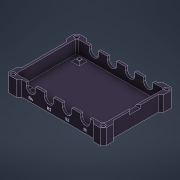
# Autodesk Inventor part: Case
Saved by Autodesk Inventor 2021.4 (Build 254397000, 397)
## iProperties
Created: 2022-02-15
Part Number: Case
Material: Generic
Document SubType Name: Modeling
Designer: Alex
Density: 1 g/cm^3
Appearance: Default
Author: Alex
Autodesk Inventor part; units mm, degrees
note: some values were not read from the file. Chosen so that the rebuilt part matches the saved one: direction of "Emboss1"; direction of "Emboss2".
ref_plane "YZ Plane" through (0, 0, 0) normal (1, 0, 0) x (0, 1, 0)
ref_plane "XZ Plane" through (0, 0, 0) normal (0, 1, 0) x (-1, 0, 0)
ref_plane "XY Plane" through (0, 0, 0) normal (0, 0, 1) x (1, 0, 0)
sketch "Sketch1" plane through (0, 0, 0) normal (0, 1, 0) x (-1, 0, 0)
  line L0 (0, -45.5) -> (-50, -45.5)
  line L1 (-50, -45.5) -> (-54, -49.5)
  line L2 (-54, -49.5) -> (-64, -49.5)
  line L3 (-64, -49.5) -> (-68, -45.5)
  line L4 (-68, -45.5) -> (-68, -35.5)
  line L5 (-68, -35.5) -> (-64, -31.5)
  line L6 (-64, -31.5) -> (-64, 0)
  line L7 (0, 0) -> (0, -45.5) construction
  line L8 (0, 0) -> (-64, 0) construction
  line L9 (0, -45.5) -> (50, -45.5)
  line L10 (50, -45.5) -> (54, -49.5)
  line L11 (54, -49.5) -> (64, -49.5)
  line L12 (64, -49.5) -> (68, -45.5)
  line L13 (68, -45.5) -> (68, -35.5)
  line L14 (68, -35.5) -> (64, -31.5)
  line L15 (64, -31.5) -> (64, 0)
  line L16 (0, 0) -> (64, 0) construction
  line L17 (0, 45.5) -> (-50, 45.5)
  line L18 (-50, 45.5) -> (-54, 49.5)
  line L19 (-54, 49.5) -> (-64, 49.5)
  line L20 (-64, 49.5) -> (-68, 45.5)
  line L21 (-68, 45.5) -> (-68, 35.5)
  line L22 (-68, 35.5) -> (-64, 31.5)
  line L23 (-64, 31.5) -> (-64, 0)
  line L24 (0, 0) -> (0, 45.5) construction
  line L25 (0, 45.5) -> (50, 45.5)
  line L26 (50, 45.5) -> (54, 49.5)
  line L27 (54, 49.5) -> (64, 49.5)
  line L28 (64, 49.5) -> (68, 45.5)
  line L29 (68, 45.5) -> (68, 35.5)
  line L30 (68, 35.5) -> (64, 31.5)
  line L31 (64, 31.5) -> (64, 0)
  dimension "d6" = 100
  dimension "d7" = 10
  dimension "d10" = 135
  dimension "d11" = 4
  dimension "d22" = 91
  constraints: 64 end point, 20 symmetric about line, 3 perpendicular, 2 horizontal, 2 horizontal alignment, 2 vertical, 2 vertical alignment
  measures "d6" diameter of L0.end L7
  measures "d7" distance of L1.end L2.end
  measures "d10" angle of L0 L1
  measures "d11" distance from line of L3.end L2
  measures "d22" distance between parallel lines of L17 L0
extrude "Extrusion1" add sketch "Sketch1" along normal blind 3
sketch "Sketch2" plane through (0, 3, 0) normal (0, 1, 0) x (1, 0, 0)
  line L0 (-61, 42.5) -> (61, 42.5)
  line L1 (61, 42.5) -> (61, -42.5)
  line L2 (61, -42.5) -> (-61, -42.5)
  line L3 (-61, -42.5) -> (-61, 42.5)
  line L4 (-54, 49.5) -> (-64, 49.5) projected
  line L5 (-64, 49.5) -> (-68, 45.5) projected
  line L6 (-68, 45.5) -> (-68, 35.5) projected
  line L7 (-68, 35.5) -> (-64, 31.5) projected
  line L8 (-64, 31.5) -> (-64, -31.5) projected
  line L9 (-64, -31.5) -> (-68, -35.5) projected
  line L10 (-68, -35.5) -> (-68, -45.5) projected
  line L11 (-68, -45.5) -> (-64, -49.5) projected
  line L12 (-64, -49.5) -> (-54, -49.5) projected
  line L13 (-54, -49.5) -> (-50, -45.5) projected
  line L14 (-50, -45.5) -> (50, -45.5) projected
  line L15 (50, -45.5) -> (54, -49.5) projected
  line L16 (54, -49.5) -> (64, -49.5) projected
  line L17 (64, -49.5) -> (68, -45.5) projected
  line L18 (68, -45.5) -> (68, -35.5) projected
  line L19 (68, -35.5) -> (64, -31.5) projected
  line L20 (64, -31.5) -> (64, 31.5) projected
  line L21 (64, 31.5) -> (68, 35.5) projected
  line L22 (68, 35.5) -> (68, 45.5) projected
  line L23 (68, 45.5) -> (64, 49.5) projected
  line L24 (64, 49.5) -> (54, 49.5) projected
  line L25 (54, 49.5) -> (50, 45.5) projected
  line L26 (50, 45.5) -> (-50, 45.5) projected
  line L27 (-50, 45.5) -> (-54, 49.5) projected
  line L28 (-49.9676, 41.5746) -> (66.2374, 41.5746) construction
  line L29 (66.2374, 41.5746) -> (66.2374, -40.9754) construction
  line L30 (66.2374, -40.9754) -> (-49.9676, -40.9754) construction
  line L31 (-49.9676, -40.9754) -> (-49.9676, 41.5746) construction
  point P0 (0, 0)
  point P1 (-61, 0)
  point P2 (0, 42.5)
  dimension "d14" = 3
  dimension "d15" = 3
  dimension "d16" = 116.205
  dimension "d17" = 82.55
  constraints: 16 end point, 3 horizontal, 3 vertical, 2 midpoint, 1 horizontal alignment, 1 vertical alignment
  measures "d14" distance between parallel lines of L26 L0
  measures "d15" distance between parallel lines of L8 L3
  measures "d16" distance of L28.start L28.end
  measures "d17" distance of L30.end L28.start
extrude "Extrusion2" add sketch "Sketch2" along normal blind 18.5
sketch "Sketch4" plane through (0, 3, 0) normal (0, 1, 0) x (1, 0, 0)
  line L0 (-56.205, 41.275) -> (60, 41.275) construction
  line L1 (60, 41.275) -> (60, -41.275) construction
  line L2 (60, -41.275) -> (-56.205, -41.275) construction
  line L3 (-56.205, -41.275) -> (-56.205, 41.275) construction
  line L4 (-61, 42.5) -> (-61, -42.5) construction
  line L5 (-61, -42.5) -> (61, -42.5) construction
  line L6 (61, -42.5) -> (61, 42.5) construction
  line L7 (61, 42.5) -> (-61, 42.5) construction
  line L8 (-64, 49.5) -> (-68, 45.5) construction
  line L9 (-68, 45.5) -> (-68, 35.5) construction
  line L10 (-68, 35.5) -> (-64, 31.5) construction
  line L11 (-64, 31.5) -> (-64, -31.5) construction
  line L12 (-64, -31.5) -> (-68, -35.5) construction
  line L13 (-68, -35.5) -> (-68, -45.5) construction
  line L14 (-68, -45.5) -> (-64, -49.5) construction
  line L15 (-64, -49.5) -> (-54, -49.5) construction
  line L16 (-54, -49.5) -> (-50, -45.5) construction
  line L17 (-50, -45.5) -> (50, -45.5) construction
  line L18 (50, -45.5) -> (54, -49.5) construction
  line L19 (54, -49.5) -> (64, -49.5) construction
  line L20 (64, -49.5) -> (68, -45.5) construction
  line L21 (68, -45.5) -> (68, -35.5) construction
  line L22 (68, -35.5) -> (64, -31.5) construction
  line L23 (64, -31.5) -> (64, 31.5) construction
  line L24 (64, 31.5) -> (68, 35.5) construction
  line L25 (68, 35.5) -> (68, 45.5) construction
  line L26 (68, 45.5) -> (64, 49.5) construction
  line L27 (64, 49.5) -> (54, 49.5) construction
  line L28 (54, 49.5) -> (50, 45.5) construction
  line L29 (50, 45.5) -> (-50, 45.5) construction
  line L30 (-50, 45.5) -> (-54, 49.5) construction
  line L31 (-54, 49.5) -> (-64, 49.5) construction
  line L32 (-61, 42.5) -> (61, 42.5) construction
  line L33 (61, 42.5) -> (61, -42.5) construction
  line L34 (61, -42.5) -> (-61, -42.5) construction
  line L35 (-61, -42.5) -> (-61, 42.5) construction
  line L36 (-52.355, 37.425) -> (-47.355, 37.425)
  line L37 (-47.355, 37.425) -> (-47.355, 32.425)
  line L38 (-47.355, 32.425) -> (-52.355, 32.425)
  line L39 (-52.355, 32.425) -> (-52.355, 37.425)
  line L40 (-52.355, 37.425) -> (-47.355, 32.425) construction
  line L41 (-47.355, 37.425) -> (-52.355, 32.425) construction
  line L42 (-52.355, -32.425) -> (-52.355, -37.425)
  line L43 (-52.355, -37.425) -> (-47.355, -37.425)
  line L44 (-47.355, -37.425) -> (-47.355, -32.425)
  line L45 (-47.355, -32.425) -> (-52.355, -32.425)
  line L46 (-52.355, -32.425) -> (-47.355, -37.425) construction
  line L47 (-52.355, -37.425) -> (-47.355, -32.425) construction
  line L48 (51.15, 37.425) -> (56.15, 37.425)
  line L49 (56.15, 37.425) -> (56.15, 32.425)
  line L50 (56.15, 32.425) -> (51.15, 32.425)
  line L51 (51.15, 32.425) -> (51.15, 37.425)
  line L52 (51.15, 37.425) -> (56.15, 32.425) construction
  line L53 (56.15, 37.425) -> (51.15, 32.425) construction
  line L54 (51.15, -32.425) -> (56.15, -32.425)
  line L55 (56.15, -32.425) -> (56.15, -37.425)
  line L56 (56.15, -37.425) -> (51.15, -37.425)
  line L57 (51.15, -37.425) -> (51.15, -32.425)
  line L58 (51.15, -32.425) -> (56.15, -37.425) construction
  line L59 (56.15, -32.425) -> (51.15, -37.425) construction
  point P0 (-61, 0)
  point P1 (-56.205, 0)
  point P2 (-49.855, 34.925)
  point P3 (-49.855, -34.925)
  point P4 (53.65, 34.925)
  point P5 (53.65, -34.925)
  point P6 (-49.855, 34.925)
  point P7 (53.65, 34.925)
  point P8 (53.65, -34.925)
  point P9 (-49.855, -34.925)
  point P10 (-49.855, 34.925)
  point P11 (-49.855, -34.925)
  point P12 (53.65, -34.925)
  point P13 (53.65, 34.925)
  dimension "d20" = 116.205
  dimension "d21" = 82.55
  dimension "d23" = 6.35
  dimension "d24" = 6.35
  dimension "d25" = 6.35
  dimension "d26" = 6.35
  dimension "d27" = 5
  dimension "d28" = 1
  constraints: 56 end point, 18 midpoint, 10 horizontal, 10 vertical, 6 equal length, 3 horizontal alignment, 2 vertical alignment, 1 point on line
  measures "d20" distance of L0.start L0.end
  measures "d21" distance of L2.end L0.start
  measures "d23" distance from line of point (-49.855, 34.925) L3
  measures "d24" distance from line of point (53.65, 34.925) L1
  measures "d25" distance from line of L0 point (-49.855, 34.925)
  measures "d26" distance from line of point (-49.855, -34.925) L2
  measures "d27" distance of L36.end L37.end
  measures "d28" distance between parallel lines of L1 L6
extrude "Extrusion3" add sketch "Sketch4" along normal blind 3
chamfer "Chamfer1" distance 3 angle 45 16 edges at (-49.855, 3, -32.425) (-47.355, 3, -34.925) (-49.855, 3, -37.425) (-52.355, 3, -34.925) (53.65, 3, -32.425) (56.15, 3, -34.925) (53.65, 3, -37.425) (51.15, 3, -34.925) (53.65, 3, 32.425) (51.15, 3, 34.925) (53.65, 3, 37.425) (56.15, 3, 34.925) (-52.355, 3, 34.925) (-49.855, 3, 32.425) (-47.355, 3, 34.925) (-49.855, 3, 37.425)
sketch "Sketch5" plane through (0, 6, 0) normal (0, 1, 0) x (1, 0, 0)
  line L0 (48.15, -29.425) -> (48.15, -40.425) construction
  line L1 (59.15, -29.425) -> (48.15, -29.425) construction
  line L2 (59.15, -40.425) -> (59.15, -29.425) construction
  line L3 (48.15, -40.425) -> (59.15, -40.425) construction
  line L4 (-44.355, 29.425) -> (-44.355, 40.425) construction
  line L5 (-55.355, 29.425) -> (-44.355, 29.425) construction
  line L6 (-55.355, 40.425) -> (-55.355, 29.425) construction
  line L7 (-44.355, 40.425) -> (-55.355, 40.425) construction
  line L8 (-61, 42.5) -> (-61, -42.5) construction
  line L9 (-61, -42.5) -> (61, -42.5) construction
  line L10 (61, -42.5) -> (61, 42.5) construction
  line L11 (61, 42.5) -> (-61, 42.5) construction
  line L12 (59.15, 29.425) -> (59.15, 40.425) construction
  line L13 (48.15, 29.425) -> (59.15, 29.425) construction
  line L14 (48.15, 40.425) -> (48.15, 29.425) construction
  line L15 (59.15, 40.425) -> (48.15, 40.425) construction
  line L16 (-55.355, -29.425) -> (-55.355, -40.425) construction
  line L17 (-44.355, -29.425) -> (-55.355, -29.425) construction
  line L18 (-44.355, -40.425) -> (-44.355, -29.425) construction
  line L19 (-55.355, -40.425) -> (-44.355, -40.425) construction
  line L20 (-52.355, 32.425) -> (-47.355, 32.425) construction
  line L21 (-47.355, 32.425) -> (-47.355, 37.425) construction
  line L22 (-47.355, 37.425) -> (-52.355, 37.425) construction
  line L23 (-52.355, 37.425) -> (-52.355, 32.425) construction
  line L24 (51.15, 32.425) -> (56.15, 32.425) construction
  line L25 (56.15, 32.425) -> (56.15, 37.425) construction
  line L26 (56.15, 37.425) -> (51.15, 37.425) construction
  line L27 (51.15, 37.425) -> (51.15, 32.425) construction
  line L28 (51.15, -37.425) -> (56.15, -37.425) construction
  line L29 (56.15, -37.425) -> (56.15, -32.425) construction
  line L30 (56.15, -32.425) -> (51.15, -32.425) construction
  line L31 (51.15, -32.425) -> (51.15, -37.425) construction
  line L32 (-52.355, -37.425) -> (-47.355, -37.425) construction
  line L33 (-47.355, -37.425) -> (-47.355, -32.425) construction
  line L34 (-47.355, -32.425) -> (-52.355, -32.425) construction
  line L35 (-52.355, -32.425) -> (-52.355, -37.425) construction
  point P0 (0, 0)
  point P1 (-49.855, 34.925)
  point P2 (53.65, 34.925)
  point P3 (53.65, -34.925)
  point P4 (-49.855, -34.925)
  point P5 (-49.855, 37.425)
  point P6 (53.65, 37.425)
  point P7 (53.65, -32.425)
  point P8 (-49.855, -32.425)
  point P9 (-47.355, -34.925)
  point P10 (-47.355, 34.925)
  point P11 (56.15, 34.925)
  point P12 (56.15, -34.925)
  constraints: 8 midpoint, 4 horizontal alignment, 4 vertical alignment
hole "Hole1" at (-49.855, 6, -34.925) at (53.65, 6, -34.925) at (53.65, 6, 34.925) at (-49.855, 6, 34.925) direction (0, -1, 0) diameter 4 depth 5
sketch "Sketch6" plane through (-50, 0, 45.5) normal (0, 0, 1) x (1, 0, 0)
  line L0 (110, 3) -> (-6.205, 3) construction
  line L1 (-5.355, 3) -> (-2.355, 6) construction
  line L2 (2.645, 6) -> (5.645, 3) construction
  line L3 (-2.355, 6) -> (2.645, 6) construction
  line L4 (98.15, 3) -> (109.15, 3) construction
  line L5 (106.15, 6) -> (109.15, 3) construction
  line L6 (101.15, 6) -> (106.15, 6) construction
  line L7 (98.15, 3) -> (101.15, 6) construction
  line L8 (106.15, 6) -> (109.15, 3) construction
  line L9 (101.15, 6) -> (106.15, 6) construction
  line L10 (98.15, 3) -> (109.15, 3) construction
  line L11 (106.15, 6) -> (109.15, 3) construction
  line L12 (101.15, 6) -> (106.15, 6) construction
  line L13 (98.15, 3) -> (101.15, 6) construction
  line L14 (-1.855, 6) -> (2.145, 6) construction
  line L15 (-6.205, 7.65) -> (110, 7.65) construction
  line L16 (110, 7.65) -> (110, 6) construction
  line L17 (110, 6) -> (-6.205, 6) construction
  line L18 (-6.205, 6) -> (-6.205, 7.65) construction
  arc A0 (6.345, 16.4) -> (19.345, 16.4) centre (12.845, 16.4) ccw
  line L19 (0, 0) -> (0, 21.5) construction
  line L20 (0, 21.5) -> (100, 21.5) construction
  line L21 (100, 0) -> (100, 21.5) construction
  line L22 (0, 0) -> (100, 0) construction
  line L23 (19.345, 16.4) -> (19.345, 21.5)
  line L24 (6.345, 16.4) -> (6.345, 21.5)
  line L25 (6.345, 21.5) -> (19.345, 21.5)
  arc A1 (19.345, 16.4) -> (6.345, 16.4) centre (12.845, 16.4) ccw construction
  arc A2 (31.745, 16.4) -> (44.745, 16.4) centre (38.245, 16.4) ccw
  arc A3 (44.745, 16.4) -> (31.745, 16.4) centre (38.245, 16.4) ccw construction
  line L26 (31.745, 16.4) -> (31.745, 21.5)
  line L27 (44.745, 16.4) -> (44.745, 21.5)
  line L28 (31.745, 21.5) -> (44.745, 21.5)
  arc A4 (57.145, 16.4) -> (70.145, 16.4) centre (63.645, 16.4) ccw
  arc A5 (70.145, 16.4) -> (57.145, 16.4) centre (63.645, 16.4) ccw construction
  line L29 (57.145, 16.4) -> (57.145, 21.5)
  line L30 (70.145, 16.4) -> (70.145, 21.5)
  line L31 (57.145, 21.5) -> (70.145, 21.5)
  arc A6 (82.545, 16.4) -> (95.545, 16.4) centre (89.045, 16.4) ccw
  arc A7 (95.545, 16.4) -> (82.545, 16.4) centre (89.045, 16.4) ccw construction
  line L32 (82.545, 16.4) -> (82.545, 21.5)
  line L33 (95.545, 16.4) -> (95.545, 21.5)
  line L34 (82.545, 21.5) -> (95.545, 21.5)
  point P0 (50, 0)
  point P1 (0.145, 3)
  dimension "d41" = 1.65
  dimension "d42" = 116.205
  dimension "d43" = 6.35
  dimension "d44" = 13
  dimension "d46" = 12.7
  dimension "d49" = 25.4
  dimension "d71" = 10.4
  constraints: 32 end point, 16 point on circle, 8 centre point, 4 horizontal, 4 vertical, 2 collinear, 2 tangent, 30 other
  measures "d41" distance of L15.end L16.end
  measures "d42" distance of L16.end L17.end
  measures "d43" distance from line of point (0.145, 3) L18
  measures "d44" diameter of A0
  measures "d46" horizontal distance of A0.centre point (0.145, 3)
  measures "d49" distance of L24.start L26.start
  measures "d71" distance from line of L17 A0.centre
extrude "Extrusion4" cut sketch "Sketch6" against normal through all
chamfer "Chamfer2" distance 2 angle 45 4 edges at (-61, 12.25, -42.5) (-61, 12.25, 42.5) (61, 12.25, 42.5) (61, 12.25, -42.5)
sketch "Sketch7" plane through (0, 21.5, 0) normal (0, 1, 0) x (1, 0, 0)
  line L0 (-43.655, -45.5) -> (-43.655, -42.5) construction
  line L1 (-43.655, -42.5) -> (-59, -42.5) construction
  line L2 (-61, -40.5) -> (-59, -42.5) construction
  line L3 (-61, -40.5) -> (-61, 40.5) construction
  line L4 (-59, 42.5) -> (-61, 40.5) construction
  line L5 (-59, 42.5) -> (-43.655, 42.5) construction
  line L6 (-43.655, 42.5) -> (-43.655, 45.5) construction
  line L7 (-43.655, 45.5) -> (-50, 45.5) construction
  line L8 (-50, 45.5) -> (-54, 49.5) construction
  line L9 (-54, 49.5) -> (-64, 49.5) construction
  line L10 (-64, 49.5) -> (-68, 45.5) construction
  line L11 (-68, 45.5) -> (-68, 35.5) construction
  line L12 (-68, 35.5) -> (-64, 31.5) construction
  line L13 (-64, 31.5) -> (-64, -31.5) construction
  line L14 (-64, -31.5) -> (-68, -35.5) construction
  line L15 (-68, -35.5) -> (-68, -45.5) construction
  line L16 (-68, -45.5) -> (-64, -49.5) construction
  line L17 (-64, -49.5) -> (-54, -49.5) construction
  line L18 (-54, -49.5) -> (-50, -45.5) construction
  line L19 (-50, -45.5) -> (-43.655, -45.5) construction
  line L20 (45.545, -42.5) -> (45.545, -45.5) construction
  line L21 (45.545, -45.5) -> (50, -45.5) construction
  line L22 (50, -45.5) -> (54, -49.5) construction
  line L23 (54, -49.5) -> (64, -49.5) construction
  line L24 (64, -49.5) -> (68, -45.5) construction
  line L25 (68, -45.5) -> (68, -35.5) construction
  line L26 (68, -35.5) -> (64, -31.5) construction
  line L27 (64, -31.5) -> (64, 31.5) construction
  line L28 (64, 31.5) -> (68, 35.5) construction
  line L29 (68, 35.5) -> (68, 45.5) construction
  line L30 (68, 45.5) -> (64, 49.5) construction
  line L31 (64, 49.5) -> (54, 49.5) construction
  line L32 (54, 49.5) -> (50, 45.5) construction
  line L33 (50, 45.5) -> (45.545, 45.5) construction
  line L34 (45.545, 45.5) -> (45.545, 42.5) construction
  line L35 (45.545, 42.5) -> (59, 42.5) construction
  line L36 (61, 40.5) -> (59, 42.5) construction
  line L37 (61, 40.5) -> (61, -40.5) construction
  line L38 (59, -42.5) -> (61, -40.5) construction
  line L39 (59, -42.5) -> (45.545, -42.5) construction
  point P0 (0, 0)
  point P1 (-63, 44.5)
  point P2 (-63, -44.5)
  point P3 (63, -44.5)
  point P4 (63, 44.5)
  dimension "d59" = 5
  dimension "d60" = 5
  dimension "d61" = 5
  dimension "d62" = 5
  constraints: 2 horizontal alignment, 2 vertical alignment
  measures "d59" distance from line of L11 point (-63, 44.5)
  measures "d60" distance from line of point (-63, 44.5) L9
  measures "d61" distance from line of point (-63, -44.5) L17
  measures "d62" distance from line of L29 point (63, 44.5)
hole "Hole2" at (-63, 21.5, -44.5) at (-63, 21.5, 44.5) at (63, 21.5, 44.5) at (63, 21.5, -44.5) direction (0, -1, 0) diameter 4 depth 6 countersink diameter 6 countersink angle 90
sketch "Sketch8" plane through (-50, 0, 45.5) normal (0, 0, 1) x (1, 0, 0)
  line L0 (10.345, 6.9) -> (15.345, 6.9) construction
  line L1 (15.345, 6.9) -> (15.345, 1.9) construction
  line L2 (15.345, 1.9) -> (10.345, 1.9) construction
  line L3 (10.345, 1.9) -> (10.345, 6.9) construction
  line L4 (35.745, 6.9) -> (40.745, 6.9) construction
  line L5 (40.745, 6.9) -> (40.745, 1.9) construction
  line L6 (40.745, 1.9) -> (35.745, 1.9) construction
  line L7 (35.745, 1.9) -> (35.745, 6.9) construction
  line L8 (61.145, 6.9) -> (66.145, 6.9) construction
  line L9 (66.145, 6.9) -> (66.145, 1.9) construction
  line L10 (66.145, 1.9) -> (61.145, 1.9) construction
  line L11 (61.145, 1.9) -> (61.145, 6.9) construction
  line L12 (86.545, 6.9) -> (91.545, 6.9) construction
  line L13 (91.545, 6.9) -> (91.545, 1.9) construction
  line L14 (91.545, 1.9) -> (86.545, 1.9) construction
  line L15 (86.545, 1.9) -> (86.545, 6.9) construction
  line L16 (57.145, 16.4) -> (57.145, 21.5) construction
  line L17 (44.745, 21.5) -> (57.145, 21.5) construction
  line L18 (44.745, 21.5) -> (44.745, 16.4) construction
  arc A0 (31.745, 16.4) -> (44.745, 16.4) centre (38.245, 16.4) ccw construction
  line L19 (31.745, 16.4) -> (31.745, 21.5) construction
  line L20 (19.345, 21.5) -> (31.745, 21.5) construction
  line L21 (19.345, 21.5) -> (19.345, 16.4) construction
  arc A1 (6.345, 16.4) -> (19.345, 16.4) centre (12.845, 16.4) ccw construction
  line L22 (6.345, 16.4) -> (6.345, 21.5) construction
  line L23 (0, 21.5) -> (6.345, 21.5) construction
  line L24 (0, 0) -> (0, 21.5) construction
  line L25 (0, 0) -> (100, 0) construction
  line L26 (100, 0) -> (100, 21.5) construction
  line L27 (95.545, 21.5) -> (100, 21.5) construction
  line L28 (95.545, 21.5) -> (95.545, 16.4) construction
  arc A2 (82.545, 16.4) -> (95.545, 16.4) centre (89.045, 16.4) ccw construction
  line L29 (82.545, 16.4) -> (82.545, 21.5) construction
  line L30 (70.145, 21.5) -> (82.545, 21.5) construction
  line L31 (70.145, 21.5) -> (70.145, 16.4) construction
  arc A3 (57.145, 16.4) -> (70.145, 16.4) centre (63.645, 16.4) ccw construction
  spline S0 degree 2 poles (12.5465, 5.1629) (12.5465, 4.6508) (12.2121, 4.396) knots 0 0 0 1 1 1
  spline S1 degree 2 poles (12.2121, 4.396) (11.9813, 4.2235) (11.7637, 4.2235) knots 0 0 0 1 1 1
  line L32 (11.7637, 4.2235) -> (11.5859, 4.2235)
  line L33 (11.5859, 4.2235) -> (12.5173, 2.9127)
  spline S2 degree 2 poles (12.5173, 2.9127) (12.5465, 2.8676) (12.5465, 2.8172) knots 0 0 0 1 1 1
  spline S3 degree 2 poles (12.5465, 2.8172) (12.5465, 2.7561) (12.451, 2.6606) (12.3899, 2.6606) knots 0 0 0 1 2 2 2
  spline S4 degree 2 poles (12.3899, 2.6606) (12.313, 2.6606) (12.2679, 2.727) knots 0 0 0 1 1 1
  line L34 (12.2679, 2.727) -> (11.1958, 4.2235)
  line L35 (11.1958, 4.2235) -> (10.4051, 4.2235)
  line L36 (10.4051, 4.2235) -> (10.4051, 2.8225)
  spline S5 degree 2 poles (10.4051, 2.8225) (10.4051, 2.6606) (10.2485, 2.6606) knots 0 0 0 1 1 1
  spline S6 degree 2 poles (10.2485, 2.6606) (10.0893, 2.6606) (10.0893, 2.8225) knots 0 0 0 1 1 1
  line L37 (10.0893, 2.8225) -> (10.0893, 6.1394)
  line L38 (10.0893, 6.1394) -> (11.5726, 6.1394)
  spline S7 degree 2 poles (11.5726, 6.1394) (11.968, 6.1394) (12.2466, 5.8846) knots 0 0 0 1 1 1
  spline S8 degree 2 poles (12.2466, 5.8846) (12.5465, 5.6113) (12.5465, 5.1629) knots 0 0 0 1 1 1
  spline S9 degree 2 poles (12.236, 5.1629) (12.236, 5.468) (12.0343, 5.6564) knots 0 0 0 1 1 1
  spline S10 degree 2 poles (12.0343, 5.6564) (11.8459, 5.8236) (11.5726, 5.8236) knots 0 0 0 1 1 1
  line L39 (11.5726, 5.8236) -> (10.4051, 5.8236)
  line L40 (10.4051, 5.8236) -> (10.4051, 4.5446)
  line L41 (10.4051, 4.5446) -> (11.7637, 4.5446)
  spline S11 degree 2 poles (11.7637, 4.5446) (11.8964, 4.5446) (12.037, 4.6667) knots 0 0 0 1 1 1
  spline S12 degree 2 poles (12.037, 4.6667) (12.236, 4.8339) (12.236, 5.1629) knots 0 0 0 1 1 1
  line L42 (15.3672, 3.2125) -> (15.0169, 3.2125)
  line L43 (15.0169, 3.2125) -> (15.0169, 2.8119)
  spline S13 degree 2 poles (15.0169, 2.8119) (15.0169, 2.65) (14.8604, 2.65) knots 0 0 0 1 1 1
  spline S14 degree 2 poles (14.8604, 2.65) (14.7011, 2.65) (14.7011, 2.8119) knots 0 0 0 1 1 1
  line L44 (14.7011, 2.8119) -> (14.7011, 3.2125)
  line L45 (14.7011, 3.2125) -> (13.1117, 3.2125)
  spline S15 degree 2 poles (13.1117, 3.2125) (13.0162, 3.2125) (13.0162, 3.3505) knots 0 0 0 1 1 1
  spline S16 degree 2 poles (13.0162, 3.3505) (13.0162, 3.4461) (13.056, 3.5575) knots 0 0 0 1 1 1
  line L46 (13.056, 3.5575) -> (13.9263, 6.0412)
  spline S17 degree 2 poles (13.9263, 6.0412) (13.9608, 6.15) (14.0669, 6.15) knots 0 0 0 1 1 1
  spline S18 degree 2 poles (14.0669, 6.15) (14.1333, 6.15) (14.2341, 6.0571) (14.2341, 5.9908) knots 0 0 0 1 2 2 2
  spline S19 degree 2 poles (14.2341, 5.9908) (14.2341, 5.9669) (14.2262, 5.9351) knots 0 0 0 1 1 1
  line L47 (14.2262, 5.9351) -> (13.3903, 3.5336)
  line L48 (13.3903, 3.5336) -> (14.7011, 3.5336)
  line L49 (14.7011, 3.5336) -> (14.7011, 4.205)
  spline S20 degree 2 poles (14.7011, 4.205) (14.7011, 4.3668) (14.8604, 4.3668) knots 0 0 0 1 1 1
  spline S21 degree 2 poles (14.8604, 4.3668) (15.0169, 4.3668) (15.0169, 4.205) knots 0 0 0 1 1 1
  line L50 (15.0169, 4.205) -> (15.0169, 3.5336)
  line L51 (15.0169, 3.5336) -> (15.3698, 3.5336)
  spline S22 degree 2 poles (15.3698, 3.5336) (15.529, 3.5336) (15.529, 3.3744) knots 0 0 0 1 1 1
  spline S23 degree 2 poles (15.529, 3.3744) (15.529, 3.2125) (15.3672, 3.2125) knots 0 0 0 1 1 1
  spline S24 degree 2 poles (37.9995, 5.2186) (37.9995, 4.7065) (37.6652, 4.4517) knots 0 0 0 1 1 1
  spline S25 degree 2 poles (37.6652, 4.4517) (37.4343, 4.2793) (37.2168, 4.2793) knots 0 0 0 1 1 1
  line L52 (37.2168, 4.2793) -> (37.039, 4.2793)
  line L53 (37.039, 4.2793) -> (37.9704, 2.9684)
  spline S26 degree 2 poles (37.9704, 2.9684) (37.9995, 2.9233) (37.9995, 2.8729) knots 0 0 0 1 1 1
  spline S27 degree 2 poles (37.9995, 2.8729) (37.9995, 2.8119) (37.904, 2.7163) (37.843, 2.7163) knots 0 0 0 1 2 2 2
  spline S28 degree 2 poles (37.843, 2.7163) (37.766, 2.7163) (37.7209, 2.7827) knots 0 0 0 1 1 1
  line L54 (37.7209, 2.7827) -> (36.6489, 4.2793)
  line L55 (36.6489, 4.2793) -> (35.8582, 4.2793)
  line L56 (35.8582, 4.2793) -> (35.8582, 2.8782)
  spline S29 degree 2 poles (35.8582, 2.8782) (35.8582, 2.7163) (35.7016, 2.7163) knots 0 0 0 1 1 1
  spline S30 degree 2 poles (35.7016, 2.7163) (35.5424, 2.7163) (35.5424, 2.8782) knots 0 0 0 1 1 1
  line L57 (35.5424, 2.8782) -> (35.5424, 6.1951)
  line L58 (35.5424, 6.1951) -> (37.0257, 6.1951)
  spline S31 degree 2 poles (37.0257, 6.1951) (37.4211, 6.1951) (37.6997, 5.9404) knots 0 0 0 1 1 1
  spline S32 degree 2 poles (37.6997, 5.9404) (37.9995, 5.6671) (37.9995, 5.2186) knots 0 0 0 1 1 1
  spline S33 degree 2 poles (37.6891, 5.2186) (37.6891, 5.5238) (37.4874, 5.7122) knots 0 0 0 1 1 1
  spline S34 degree 2 poles (37.4874, 5.7122) (37.299, 5.8793) (37.0257, 5.8793) knots 0 0 0 1 1 1
  line L59 (37.0257, 5.8793) -> (35.8582, 5.8793)
  line L60 (35.8582, 5.8793) -> (35.8582, 4.6003)
  line L61 (35.8582, 4.6003) -> (37.2168, 4.6003)
  spline S35 degree 2 poles (37.2168, 4.6003) (37.3494, 4.6003) (37.4901, 4.7224) knots 0 0 0 1 1 1
  spline S36 degree 2 poles (37.4901, 4.7224) (37.6891, 4.8896) (37.6891, 5.2186) knots 0 0 0 1 1 1
  spline S37 degree 2 poles (40.7539, 3.9502) (40.7539, 3.263) (40.2816, 2.918) knots 0 0 0 1 1 1
  spline S38 degree 2 poles (40.2816, 2.918) (39.8384, 2.5996) (39.321, 2.7561) knots 0 0 0 1 1 1
  spline S39 degree 2 poles (39.321, 2.7561) (38.7744, 2.9233) (38.5807, 3.523) knots 0 0 0 1 1 1
  spline S40 degree 2 poles (38.5807, 3.523) (38.5701, 3.5549) (38.5701, 3.5787) knots 0 0 0 1 1 1
  spline S41 degree 2 poles (38.5701, 3.5787) (38.5701, 3.7273) (38.7266, 3.7273) knots 0 0 0 1 1 1
  spline S42 degree 2 poles (38.7266, 3.7273) (38.8354, 3.7273) (38.8699, 3.6185) knots 0 0 0 1 1 1
  spline S43 degree 2 poles (38.8699, 3.6185) (38.9601, 3.3346) (39.1804, 3.1834) knots 0 0 0 1 1 1
  spline S44 degree 2 poles (39.1804, 3.1834) (39.3767, 3.0401) (39.6262, 3.0401) knots 0 0 0 1 1 1
  spline S45 degree 2 poles (39.6262, 3.0401) (39.9552, 3.0401) (40.1887, 3.2736) knots 0 0 0 1 1 1
  spline S46 degree 2 poles (40.1887, 3.2736) (40.4488, 3.5283) (40.4488, 3.9502) knots 0 0 0 1 1 1
  spline S47 degree 2 poles (40.4488, 3.9502) (40.4488, 4.3907) (40.1861, 4.6189) knots 0 0 0 1 1 1
  spline S48 degree 2 poles (40.1861, 4.6189) (39.9923, 4.7887) (39.666, 4.8392) knots 0 0 0 1 1 1
  spline S49 degree 2 poles (39.666, 4.8392) (39.4935, 4.8498) (39.1591, 4.8843) (39.1591, 4.9745) knots 0 0 0 1 2 2 2
  spline S50 degree 2 poles (39.1591, 4.9745) (39.1591, 5.0567) (39.2361, 5.1337) knots 0 0 0 1 1 1
  line L62 (39.2361, 5.1337) -> (39.9711, 5.8793)
  line L63 (39.9711, 5.8793) -> (38.8858, 5.8793)
  spline S51 degree 2 poles (38.8858, 5.8793) (38.7266, 5.8793) (38.7266, 6.0386) knots 0 0 0 1 1 1
  spline S52 degree 2 poles (38.7266, 6.0386) (38.7266, 6.1951) (38.8858, 6.1951) knots 0 0 0 1 1 1
  line L64 (38.8858, 6.1951) -> (40.4434, 6.2004)
  spline S53 degree 2 poles (40.4434, 6.2004) (40.5655, 6.2004) (40.5655, 6.1208) knots 0 0 0 1 1 1
  spline S54 degree 2 poles (40.5655, 6.1208) (40.5655, 6.0545) (40.4169, 5.9032) knots 0 0 0 1 1 1
  line L65 (40.4169, 5.9032) -> (39.7031, 5.1629)
  spline S55 degree 2 poles (39.7031, 5.1629) (40.7539, 5.0223) (40.7539, 3.9502) knots 0 0 0 1 1 1
  spline S56 degree 2 poles (63.4526, 5.1456) (63.4526, 4.6335) (63.1183, 4.3788) knots 0 0 0 1 1 1
  spline S57 degree 2 poles (63.1183, 4.3788) (62.8874, 4.2063) (62.6698, 4.2063) knots 0 0 0 1 1 1
  line L66 (62.6698, 4.2063) -> (62.492, 4.2063)
  line L67 (62.492, 4.2063) -> (63.4234, 2.8955)
  spline S58 degree 2 poles (63.4234, 2.8955) (63.4526, 2.8503) (63.4526, 2.7999) knots 0 0 0 1 1 1
  spline S59 degree 2 poles (63.4526, 2.7999) (63.4526, 2.7389) (63.3571, 2.6434) (63.2961, 2.6434) knots 0 0 0 1 2 2 2
  spline S60 degree 2 poles (63.2961, 2.6434) (63.2191, 2.6434) (63.174, 2.7097) knots 0 0 0 1 1 1
  line L68 (63.174, 2.7097) -> (62.102, 4.2063)
  line L69 (62.102, 4.2063) -> (61.3112, 4.2063)
  line L70 (61.3112, 4.2063) -> (61.3112, 2.8052)
  spline S61 degree 2 poles (61.3112, 2.8052) (61.3112, 2.6434) (61.1547, 2.6434) knots 0 0 0 1 1 1
  spline S62 degree 2 poles (61.1547, 2.6434) (60.9955, 2.6434) (60.9955, 2.8052) knots 0 0 0 1 1 1
  line L71 (60.9955, 2.8052) -> (60.9955, 6.1221)
  line L72 (60.9955, 6.1221) -> (62.4788, 6.1221)
  spline S63 degree 2 poles (62.4788, 6.1221) (62.8742, 6.1221) (63.1528, 5.8674) knots 0 0 0 1 1 1
  spline S64 degree 2 poles (63.1528, 5.8674) (63.4526, 5.5941) (63.4526, 5.1456) knots 0 0 0 1 1 1
  spline S65 degree 2 poles (63.1422, 5.1456) (63.1422, 5.4508) (62.9405, 5.6392) knots 0 0 0 1 1 1
  spline S66 degree 2 poles (62.9405, 5.6392) (62.7521, 5.8064) (62.4788, 5.8064) knots 0 0 0 1 1 1
  line L73 (62.4788, 5.8064) -> (61.3112, 5.8064)
  line L74 (61.3112, 5.8064) -> (61.3112, 4.5274)
  line L75 (61.3112, 4.5274) -> (62.6698, 4.5274)
  spline S67 degree 2 poles (62.6698, 4.5274) (62.8025, 4.5274) (62.9431, 4.6494) knots 0 0 0 1 1 1
  spline S68 degree 2 poles (62.9431, 4.6494) (63.1422, 4.8166) (63.1422, 5.1456) knots 0 0 0 1 1 1
  line L76 (65.9629, 2.6885) -> (64.0284, 2.6885)
  spline S69 degree 2 poles (64.0284, 2.6885) (64.116, 3.0096) (64.2009, 3.3227) knots 0 0 0 1 1 1
  spline S70 degree 2 poles (64.2009, 3.3227) (64.3389, 3.7499) (64.583, 4.063) knots 0 0 0 1 1 1
  spline S71 degree 2 poles (64.583, 4.063) (64.9068, 4.4796) (65.4773, 4.8007) knots 0 0 0 1 1 1
  spline S72 degree 2 poles (65.4773, 4.8007) (65.8222, 4.9917) (65.8222, 5.3287) knots 0 0 0 1 1 1
  spline S73 degree 2 poles (65.8222, 5.3287) (65.8222, 5.5357) (65.6736, 5.6843) knots 0 0 0 1 1 1
  spline S74 degree 2 poles (65.6736, 5.6843) (65.5118, 5.8356) (65.2491, 5.8356) knots 0 0 0 1 1 1
  spline S75 degree 2 poles (65.2491, 5.8356) (64.9572, 5.8356) (64.7953, 5.7506) knots 0 0 0 1 1 1
  spline S76 degree 2 poles (64.7953, 5.7506) (64.6069, 5.6418) (64.4955, 5.3685) knots 0 0 0 1 1 1
  spline S77 degree 2 poles (64.4955, 5.3685) (64.4557, 5.273) (64.3628, 5.273) knots 0 0 0 1 1 1
  spline S78 degree 2 poles (64.3628, 5.273) (64.2062, 5.273) (64.2062, 5.4269) knots 0 0 0 1 1 1
  spline S79 degree 2 poles (64.2062, 5.4269) (64.2062, 5.4561) (64.2221, 5.4906) knots 0 0 0 1 1 1
  spline S80 degree 2 poles (64.2221, 5.4906) (64.4955, 6.1566) (65.2278, 6.1566) knots 0 0 0 1 1 1
  spline S81 degree 2 poles (65.2278, 6.1566) (65.6577, 6.1566) (65.9177, 5.9125) knots 0 0 0 1 1 1
  spline S82 degree 2 poles (65.9177, 5.9125) (66.1566, 5.6896) (66.1566, 5.3553) knots 0 0 0 1 1 1
  spline S83 degree 2 poles (66.1566, 5.3553) (66.1566, 4.8325) (65.6232, 4.5274) knots 0 0 0 1 1 1
  spline S84 degree 2 poles (65.6232, 4.5274) (64.9996, 4.1718) (64.7184, 3.7154) knots 0 0 0 1 1 1
  spline S85 degree 2 poles (64.7184, 3.7154) (64.583, 3.4872) (64.4503, 3.0042) knots 0 0 0 1 1 1
  line L77 (64.4503, 3.0042) -> (65.9629, 3.0042)
  spline S86 degree 2 poles (65.9629, 3.0042) (66.1221, 3.0042) (66.1221, 2.8477) knots 0 0 0 1 1 1
  spline S87 degree 2 poles (66.1221, 2.8477) (66.1221, 2.6885) (65.9629, 2.6885) knots 0 0 0 1 1 1
  spline S88 degree 2 poles (89.4775, 5.1602) (89.4775, 4.6481) (89.1432, 4.3934) knots 0 0 0 1 1 1
  spline S89 degree 2 poles (89.1432, 4.3934) (88.9123, 4.2209) (88.6947, 4.2209) knots 0 0 0 1 1 1
  line L78 (88.6947, 4.2209) -> (88.5169, 4.2209)
  line L79 (88.5169, 4.2209) -> (89.4483, 2.91)
  spline S90 degree 2 poles (89.4483, 2.91) (89.4775, 2.8649) (89.4775, 2.8145) knots 0 0 0 1 1 1
  spline S91 degree 2 poles (89.4775, 2.8145) (89.4775, 2.7535) (89.382, 2.658) (89.321, 2.658) knots 0 0 0 1 2 2 2
  spline S92 degree 2 poles (89.321, 2.658) (89.244, 2.658) (89.1989, 2.7243) knots 0 0 0 1 1 1
  line L80 (89.1989, 2.7243) -> (88.1269, 4.2209)
  line L81 (88.1269, 4.2209) -> (87.3361, 4.2209)
  line L82 (87.3361, 4.2209) -> (87.3361, 2.8198)
  spline S93 degree 2 poles (87.3361, 2.8198) (87.3361, 2.658) (87.1796, 2.658) knots 0 0 0 1 1 1
  spline S94 degree 2 poles (87.1796, 2.658) (87.0204, 2.658) (87.0204, 2.8198) knots 0 0 0 1 1 1
  line L83 (87.0204, 2.8198) -> (87.0204, 6.1367)
  line L84 (87.0204, 6.1367) -> (88.5037, 6.1367)
  spline S95 degree 2 poles (88.5037, 6.1367) (88.8991, 6.1367) (89.1777, 5.882) knots 0 0 0 1 1 1
  spline S96 degree 2 poles (89.1777, 5.882) (89.4775, 5.6087) (89.4775, 5.1602) knots 0 0 0 1 1 1
  spline S97 degree 2 poles (89.1671, 5.1602) (89.1671, 5.4654) (88.9654, 5.6538) knots 0 0 0 1 1 1
  spline S98 degree 2 poles (88.9654, 5.6538) (88.777, 5.821) (88.5037, 5.821) knots 0 0 0 1 1 1
  line L85 (88.5037, 5.821) -> (87.3361, 5.821)
  line L86 (87.3361, 5.821) -> (87.3361, 4.542)
  line L87 (87.3361, 4.542) -> (88.6947, 4.542)
  spline S99 degree 2 poles (88.6947, 4.542) (88.8274, 4.542) (88.968, 4.664) knots 0 0 0 1 1 1
  spline S100 degree 2 poles (88.968, 4.664) (89.1671, 4.8312) (89.1671, 5.1602) knots 0 0 0 1 1 1
  spline S101 degree 2 poles (90.6928, 2.8145) (90.6928, 2.658) (90.5389, 2.658) knots 0 0 0 1 1 1
  spline S102 degree 2 poles (90.5389, 2.658) (90.3824, 2.658) (90.3824, 2.8145) knots 0 0 0 1 1 1
  line L88 (90.3824, 2.8145) -> (90.3824, 5.9855)
  spline S103 degree 2 poles (90.3824, 5.9855) (90.3824, 6.142) (90.5389, 6.142) knots 0 0 0 1 1 1
  spline S104 degree 2 poles (90.5389, 6.142) (90.6928, 6.142) (90.6928, 5.9855) knots 0 0 0 1 1 1
  line L89 (90.6928, 5.9855) -> (90.6928, 2.8145)
  point P0 (50, 0)
  point P1 (38.245, 9.9)
  point P2 (38.245, 6.9)
  point P3 (63.645, 6.9)
  point P4 (63.645, 9.9)
  point P5 (89.045, 6.9)
  point P6 (89.045, 9.9)
  point P7 (12.845, 9.9)
  point P8 (12.845, 6.9)
  point P9 (15.345, 4.4)
  dimension "d72" = 5
  dimension "d74" = 3
  constraints: 6 collinear, 5 midpoint, 5 vertical alignment, 4 equal length, 4 point on circle, 1 horizontal, 8 other
  measures "d72" distance of L1.end L2.end
  measures "d74" distance of point (12.845, 6.9) point (12.845, 9.9)
emboss "Emboss1" sketch "Sketch8" operation cut depth 1 direction (0, 0, -1)
sketch "Sketch9" plane through (50, 0, -45.5) normal (0, 0, -1) x (-1, 0, 0)
  line L0 (42.855, 21.5) -> (42.855, 16.4) construction
  arc A0 (29.855, 16.4) -> (42.855, 16.4) centre (36.355, 16.4) ccw construction
  line L1 (29.855, 16.4) -> (29.855, 21.5) construction
  line L2 (17.455, 21.5) -> (29.855, 21.5) construction
  line L3 (17.455, 21.5) -> (17.455, 16.4) construction
  arc A1 (4.455, 16.4) -> (17.455, 16.4) centre (10.955, 16.4) ccw construction
  line L4 (4.455, 16.4) -> (4.455, 21.5) construction
  line L5 (0, 21.5) -> (4.455, 21.5) construction
  line L6 (0, 0) -> (0, 21.5) construction
  line L7 (0, 0) -> (100, 0) construction
  line L8 (100, 0) -> (100, 21.5) construction
  line L9 (93.655, 21.5) -> (100, 21.5) construction
  line L10 (93.655, 21.5) -> (93.655, 16.4) construction
  arc A2 (80.655, 16.4) -> (93.655, 16.4) centre (87.155, 16.4) ccw construction
  line L11 (80.655, 16.4) -> (80.655, 21.5) construction
  line L12 (68.255, 21.5) -> (80.655, 21.5) construction
  line L13 (68.255, 21.5) -> (68.255, 16.4) construction
  arc A3 (55.255, 16.4) -> (68.255, 16.4) centre (61.755, 16.4) ccw construction
  line L14 (55.255, 16.4) -> (55.255, 21.5) construction
  line L15 (42.855, 21.5) -> (55.255, 21.5) construction
  line L16 (8.455, 6.9) -> (13.455, 6.9) construction
  line L17 (13.455, 6.9) -> (13.455, 1.9) construction
  line L18 (13.455, 1.9) -> (8.455, 1.9) construction
  line L19 (8.455, 1.9) -> (8.455, 6.9) construction
  line L20 (33.855, 6.9) -> (38.855, 6.9) construction
  line L21 (38.855, 6.9) -> (38.855, 1.9) construction
  line L22 (38.855, 1.9) -> (33.855, 1.9) construction
  line L23 (33.855, 1.9) -> (33.855, 6.9) construction
  line L24 (59.255, 6.9) -> (64.255, 6.9) construction
  line L25 (64.255, 6.9) -> (64.255, 1.9) construction
  line L26 (64.255, 1.9) -> (59.255, 1.9) construction
  line L27 (59.255, 1.9) -> (59.255, 6.9) construction
  line L28 (84.655, 6.9) -> (89.655, 6.9) construction
  line L29 (89.655, 6.9) -> (89.655, 1.9) construction
  line L30 (89.655, 1.9) -> (84.655, 1.9) construction
  line L31 (84.655, 1.9) -> (84.655, 6.9) construction
  line L32 (11.1633, 2.6978) -> (9.0352, 2.6978)
  line L33 (9.0352, 2.6978) -> (9.0352, 5.9802)
  spline S0 degree 2 poles (9.0352, 5.9802) (9.0352, 6.142) (9.1917, 6.142) knots 0 0 0 1 1 1
  spline S1 degree 2 poles (9.1917, 6.142) (9.3456, 6.142) (9.3456, 5.9802) knots 0 0 0 1 1 1
  line L34 (9.3456, 5.9802) -> (9.3456, 3.0135)
  line L35 (9.3456, 3.0135) -> (11.1633, 3.0135)
  spline S2 degree 2 poles (11.1633, 3.0135) (11.3199, 3.0135) (11.3199, 2.857) knots 0 0 0 1 1 1
  spline S3 degree 2 poles (11.3199, 2.857) (11.3199, 2.6978) (11.1633, 2.6978) knots 0 0 0 1 1 1
  spline S4 degree 2 poles (12.5033, 2.8145) (12.5033, 2.658) (12.3494, 2.658) knots 0 0 0 1 1 1
  spline S5 degree 2 poles (12.3494, 2.658) (12.1929, 2.658) (12.1929, 2.8145) knots 0 0 0 1 1 1
  line L36 (12.1929, 2.8145) -> (12.1929, 5.9855)
  spline S6 degree 2 poles (12.1929, 5.9855) (12.1929, 6.142) (12.3494, 6.142) knots 0 0 0 1 1 1
  spline S7 degree 2 poles (12.3494, 6.142) (12.5033, 6.142) (12.5033, 5.9855) knots 0 0 0 1 1 1
  line L37 (12.5033, 5.9855) -> (12.5033, 2.8145)
  line L38 (35.9384, 2.6633) -> (33.8103, 2.6633)
  line L39 (33.8103, 2.6633) -> (33.8103, 5.9457)
  spline S8 degree 2 poles (33.8103, 5.9457) (33.8103, 6.1075) (33.9668, 6.1075) knots 0 0 0 1 1 1
  spline S9 degree 2 poles (33.9668, 6.1075) (34.1207, 6.1075) (34.1207, 5.9457) knots 0 0 0 1 1 1
  line L40 (34.1207, 5.9457) -> (34.1207, 2.979)
  line L41 (34.1207, 2.979) -> (35.9384, 2.979)
  spline S10 degree 2 poles (35.9384, 2.979) (36.095, 2.979) (36.095, 2.8225) knots 0 0 0 1 1 1
  spline S11 degree 2 poles (36.095, 2.8225) (36.095, 2.6633) (35.9384, 2.6633) knots 0 0 0 1 1 1
  line L42 (38.5733, 2.6686) -> (36.6389, 2.6686)
  spline S12 degree 2 poles (36.6389, 2.6686) (36.7265, 2.9897) (36.8114, 3.3028) knots 0 0 0 1 1 1
  spline S13 degree 2 poles (36.8114, 3.3028) (36.9494, 3.73) (37.1935, 4.0431) knots 0 0 0 1 1 1
  spline S14 degree 2 poles (37.1935, 4.0431) (37.5172, 4.4597) (38.0878, 4.7808) knots 0 0 0 1 1 1
  spline S15 degree 2 poles (38.0878, 4.7808) (38.4327, 4.9718) (38.4327, 5.3088) knots 0 0 0 1 1 1
  spline S16 degree 2 poles (38.4327, 5.3088) (38.4327, 5.5158) (38.2841, 5.6644) knots 0 0 0 1 1 1
  spline S17 degree 2 poles (38.2841, 5.6644) (38.1222, 5.8157) (37.8595, 5.8157) knots 0 0 0 1 1 1
  spline S18 degree 2 poles (37.8595, 5.8157) (37.5677, 5.8157) (37.4058, 5.7307) knots 0 0 0 1 1 1
  spline S19 degree 2 poles (37.4058, 5.7307) (37.2174, 5.6219) (37.1059, 5.3486) knots 0 0 0 1 1 1
  spline S20 degree 2 poles (37.1059, 5.3486) (37.0661, 5.2531) (36.9733, 5.2531) knots 0 0 0 1 1 1
  spline S21 degree 2 poles (36.9733, 5.2531) (36.8167, 5.2531) (36.8167, 5.407) knots 0 0 0 1 1 1
  spline S22 degree 2 poles (36.8167, 5.407) (36.8167, 5.4362) (36.8326, 5.4707) knots 0 0 0 1 1 1
  spline S23 degree 2 poles (36.8326, 5.4707) (37.1059, 6.1367) (37.8383, 6.1367) knots 0 0 0 1 1 1
  spline S24 degree 2 poles (37.8383, 6.1367) (38.2682, 6.1367) (38.5282, 5.8926) knots 0 0 0 1 1 1
  spline S25 degree 2 poles (38.5282, 5.8926) (38.7671, 5.6697) (38.7671, 5.3354) knots 0 0 0 1 1 1
  spline S26 degree 2 poles (38.7671, 5.3354) (38.7671, 4.8126) (38.2337, 4.5075) knots 0 0 0 1 1 1
  spline S27 degree 2 poles (38.2337, 4.5075) (37.6101, 4.1519) (37.3288, 3.6955) knots 0 0 0 1 1 1
  spline S28 degree 2 poles (37.3288, 3.6955) (37.1935, 3.4673) (37.0608, 2.9843) knots 0 0 0 1 1 1
  line L43 (37.0608, 2.9843) -> (38.5733, 2.9843)
  spline S29 degree 2 poles (38.5733, 2.9843) (38.7326, 2.9843) (38.7326, 2.8278) knots 0 0 0 1 1 1
  spline S30 degree 2 poles (38.7326, 2.8278) (38.7326, 2.6686) (38.5733, 2.6686) knots 0 0 0 1 1 1
  line L44 (61.2853, 2.7561) -> (59.1572, 2.7561)
  line L45 (59.1572, 2.7561) -> (59.1572, 6.0386)
  spline S31 degree 2 poles (59.1572, 6.0386) (59.1572, 6.2004) (59.3138, 6.2004) knots 0 0 0 1 1 1
  spline S32 degree 2 poles (59.3138, 6.2004) (59.4677, 6.2004) (59.4677, 6.0386) knots 0 0 0 1 1 1
  line L46 (59.4677, 6.0386) -> (59.4677, 3.0719)
  line L47 (59.4677, 3.0719) -> (61.2853, 3.0719)
  spline S33 degree 2 poles (61.2853, 3.0719) (61.4419, 3.0719) (61.4419, 2.9154) knots 0 0 0 1 1 1
  spline S34 degree 2 poles (61.4419, 2.9154) (61.4419, 2.7561) (61.2853, 2.7561) knots 0 0 0 1 1 1
  spline S35 degree 2 poles (64.1644, 3.9502) (64.1644, 3.263) (63.6921, 2.918) knots 0 0 0 1 1 1
  spline S36 degree 2 poles (63.6921, 2.918) (63.2489, 2.5996) (62.7315, 2.7561) knots 0 0 0 1 1 1
  spline S37 degree 2 poles (62.7315, 2.7561) (62.1849, 2.9233) (61.9912, 3.523) knots 0 0 0 1 1 1
  spline S38 degree 2 poles (61.9912, 3.523) (61.9805, 3.5549) (61.9805, 3.5787) knots 0 0 0 1 1 1
  spline S39 degree 2 poles (61.9805, 3.5787) (61.9805, 3.7273) (62.1371, 3.7273) knots 0 0 0 1 1 1
  spline S40 degree 2 poles (62.1371, 3.7273) (62.2459, 3.7273) (62.2804, 3.6185) knots 0 0 0 1 1 1
  spline S41 degree 2 poles (62.2804, 3.6185) (62.3706, 3.3346) (62.5909, 3.1834) knots 0 0 0 1 1 1
  spline S42 degree 2 poles (62.5909, 3.1834) (62.7872, 3.0401) (63.0367, 3.0401) knots 0 0 0 1 1 1
  spline S43 degree 2 poles (63.0367, 3.0401) (63.3657, 3.0401) (63.5992, 3.2736) knots 0 0 0 1 1 1
  spline S44 degree 2 poles (63.5992, 3.2736) (63.8592, 3.5283) (63.8592, 3.9502) knots 0 0 0 1 1 1
  spline S45 degree 2 poles (63.8592, 3.9502) (63.8592, 4.3907) (63.5965, 4.6189) knots 0 0 0 1 1 1
  spline S46 degree 2 poles (63.5965, 4.6189) (63.4028, 4.7887) (63.0765, 4.8392) knots 0 0 0 1 1 1
  spline S47 degree 2 poles (63.0765, 4.8392) (62.904, 4.8498) (62.5696, 4.8843) (62.5696, 4.9745) knots 0 0 0 1 2 2 2
  spline S48 degree 2 poles (62.5696, 4.9745) (62.5696, 5.0567) (62.6466, 5.1337) knots 0 0 0 1 1 1
  line L48 (62.6466, 5.1337) -> (63.3816, 5.8793)
  line L49 (63.3816, 5.8793) -> (62.2963, 5.8793)
  spline S49 degree 2 poles (62.2963, 5.8793) (62.1371, 5.8793) (62.1371, 6.0386) knots 0 0 0 1 1 1
  spline S50 degree 2 poles (62.1371, 6.0386) (62.1371, 6.1951) (62.2963, 6.1951) knots 0 0 0 1 1 1
  line L50 (62.2963, 6.1951) -> (63.8539, 6.2004)
  spline S51 degree 2 poles (63.8539, 6.2004) (63.976, 6.2004) (63.976, 6.1208) knots 0 0 0 1 1 1
  spline S52 degree 2 poles (63.976, 6.1208) (63.976, 6.0545) (63.8274, 5.9032) knots 0 0 0 1 1 1
  line L51 (63.8274, 5.9032) -> (63.1136, 5.1629)
  spline S53 degree 2 poles (63.1136, 5.1629) (64.1644, 5.0223) (64.1644, 3.9502) knots 0 0 0 1 1 1
  line L52 (86.6323, 2.7004) -> (84.5041, 2.7004)
  line L53 (84.5041, 2.7004) -> (84.5041, 5.9828)
  spline S54 degree 2 poles (84.5041, 5.9828) (84.5041, 6.1447) (84.6607, 6.1447) knots 0 0 0 1 1 1
  spline S55 degree 2 poles (84.6607, 6.1447) (84.8146, 6.1447) (84.8146, 5.9828) knots 0 0 0 1 1 1
  line L54 (84.8146, 5.9828) -> (84.8146, 3.0162)
  line L55 (84.8146, 3.0162) -> (86.6323, 3.0162)
  spline S56 degree 2 poles (86.6323, 3.0162) (86.7888, 3.0162) (86.7888, 2.8596) knots 0 0 0 1 1 1
  spline S57 degree 2 poles (86.7888, 2.8596) (86.7888, 2.7004) (86.6323, 2.7004) knots 0 0 0 1 1 1
  line L56 (89.5777, 3.2125) -> (89.2274, 3.2125)
  line L57 (89.2274, 3.2125) -> (89.2274, 2.8119)
  spline S58 degree 2 poles (89.2274, 2.8119) (89.2274, 2.65) (89.0708, 2.65) knots 0 0 0 1 1 1
  spline S59 degree 2 poles (89.0708, 2.65) (88.9116, 2.65) (88.9116, 2.8119) knots 0 0 0 1 1 1
  line L58 (88.9116, 2.8119) -> (88.9116, 3.2125)
  line L59 (88.9116, 3.2125) -> (87.3222, 3.2125)
  spline S60 degree 2 poles (87.3222, 3.2125) (87.2266, 3.2125) (87.2266, 3.3505) knots 0 0 0 1 1 1
  spline S61 degree 2 poles (87.2266, 3.3505) (87.2266, 3.4461) (87.2664, 3.5575) knots 0 0 0 1 1 1
  line L60 (87.2664, 3.5575) -> (88.1368, 6.0412)
  spline S62 degree 2 poles (88.1368, 6.0412) (88.1713, 6.15) (88.2774, 6.15) knots 0 0 0 1 1 1
  spline S63 degree 2 poles (88.2774, 6.15) (88.3438, 6.15) (88.4446, 6.0571) (88.4446, 5.9908) knots 0 0 0 1 2 2 2
  spline S64 degree 2 poles (88.4446, 5.9908) (88.4446, 5.9669) (88.4367, 5.9351) knots 0 0 0 1 1 1
  line L61 (88.4367, 5.9351) -> (87.6008, 3.5336)
  line L62 (87.6008, 3.5336) -> (88.9116, 3.5336)
  line L63 (88.9116, 3.5336) -> (88.9116, 4.205)
  spline S65 degree 2 poles (88.9116, 4.205) (88.9116, 4.3668) (89.0708, 4.3668) knots 0 0 0 1 1 1
  spline S66 degree 2 poles (89.0708, 4.3668) (89.2274, 4.3668) (89.2274, 4.205) knots 0 0 0 1 1 1
  line L64 (89.2274, 4.205) -> (89.2274, 3.5336)
  line L65 (89.2274, 3.5336) -> (89.5803, 3.5336)
  spline S67 degree 2 poles (89.5803, 3.5336) (89.7395, 3.5336) (89.7395, 3.3744) knots 0 0 0 1 1 1
  spline S68 degree 2 poles (89.7395, 3.3744) (89.7395, 3.2125) (89.5777, 3.2125) knots 0 0 0 1 1 1
  point P0 (50, 0)
  point P1 (10.955, 6.9)
  point P2 (10.955, 9.9)
  point P3 (36.355, 6.9)
  point P4 (36.355, 9.9)
  point P5 (61.755, 6.9)
  point P6 (61.755, 9.9)
  point P7 (87.155, 6.9)
  point P8 (87.155, 9.9)
  dimension "d77" = 5
  dimension "d79" = 3
  constraints: 7 equal length, 6 collinear, 4 midpoint, 4 point on circle, 4 vertical alignment, 1 horizontal, 8 other
  measures "d77" distance of L18.end L16.start
  measures "d79" distance from line of L16 point (10.955, 9.9)
emboss "Emboss2" sketch "Sketch9" operation cut depth 1 direction (0, 0, 1)
sketch "Sketch10" plane through (64, 0, 31.5) normal (1, 0, 0) x (0, 0, -1)
  line L0 (0, 0) -> (63, 0) construction
  line L1 (63, 0) -> (63, 21.5) construction
  line L2 (0, 21.5) -> (63, 21.5) construction
  line L3 (0, 0) -> (0, 21.5) construction
  line L4 (72, 3) -> (72, 21.5) construction
  line L5 (-9, 3) -> (72, 3) construction
  line L6 (-9, 21.5) -> (-9, 3) construction
  line L7 (72, 21.5) -> (-9, 21.5) construction
  line L8 (-8.925, 3) -> (2.075, 3) construction
  line L9 (-0.925, 6) -> (2.075, 3) construction
  line L10 (-5.925, 6) -> (-0.925, 6) construction
  line L11 (-5.925, 6) -> (-8.925, 3) construction
  line L12 (63.925, 6) -> (68.925, 6) construction
  line L13 (63.925, 6) -> (60.925, 3) construction
  line L14 (60.925, 3) -> (71.925, 3) construction
  line L15 (68.925, 6) -> (71.925, 3) construction
  line L16 (25.725, 25) -> (34.725, 25)
  line L17 (34.725, 25) -> (34.725, 20)
  line L18 (34.725, 20) -> (25.725, 20)
  line L19 (25.725, 20) -> (25.725, 25)
  point P0 (31.5, 0)
  point P1 (-9.775, 3)
  point P2 (-9.775, 3)
  point P3 (-9.775, 3)
  dimension "d83" = 5
  dimension "d84" = 14
  dimension "d85" = 9
  dimension "d86" = 35.5
  constraints: 8 end point, 2 vertical, 1 horizontal
  measures "d83" distance of L16.end L17.end
  measures "d84" distance between parallel lines of L18 L10
  measures "d85" distance of L16.start L16.end
  measures "d86" distance from line of L19 point (-9.775, 3)
extrude "Extrusion5" cut sketch "Sketch10" against normal blind 10
chamfer "Chamfer3" distance 3 angle 45 3 edges at (64, 20, 1.275) (64, 20.75, 5.775) (64, 20.75, -3.225)
equation "\"d15\" = d14"
equation "\"d24\" = d23"
equation "\"d25\" = d23"
equation "\"d26\" = d23"
body "Solid1"
